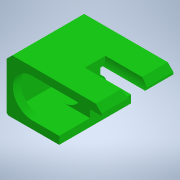
# Autodesk Inventor part: Y-linear bearing shroud secondary
Saved by Autodesk Inventor 2020.4 (Build 244396000, 396)
## iProperties
Created: 2021-02-25
Part Number: Y-linear bearing shroud secondary
Material: ABS Plastic
Document SubType Name: Modeling
Designer: AOB
Mass: 6.2455 g
Surface Area: 48.8239 cm^2
Volume: 5.89199 cm^3
Density: 1.06 g/cm^3
Appearance: Dark Green
Author: AOB
Autodesk Inventor part; units mm, degrees
ref_plane "YZ Plane" through (0, 0, 0) normal (1, 0, 0) x (0, 1, 0)
ref_plane "XZ Plane" through (0, 0, 0) normal (0, 1, 0) x (-1, 0, 0)
sketch "Sketch1" plane through (0, 0, 0) normal (0, 0, 1) x (1, 0, 0)
  line L0 (-9.0445, -10.4807) -> (0.0261, -10.458)
  line L1 (-10, 8.3388) -> (-10, 0)
  line L2 (-10, 0) -> (-9.9763, -9.4855)
  line L3 (27, 8.3389) -> (27, 7.5575)
  line L4 (24.782, 10.5568) -> (27, 8.3389)
  line L5 (-7.782, 10.5568) -> (-10, 8.3388)
  arc A0 (-9.9763, -9.4855) -> (-8.9738, -10.483) centre (-8.9763, -9.483) ccw
  arc A1 (-0.0188, 7.5552) -> (-0.012, -7.4448) centre (-0.0154, 0.0552) ccw
  line L6 (5, 7.5575) -> (-0.0188, 7.5552)
  line L7 (0.0261, -10.458) -> (7.5, -10.458)
  line L8 (7.5, 0.0187) -> (10.5, 0.0187) construction
  line L9 (10.5, -10.458) -> (7.5, -10.458)
  line L10 (-0.012, -7.4448) -> (10.5, -7.4448)
  line L11 (10.5, -7.4448) -> (10.5, -10.458)
  line L12 (-7.782, 10.5568) -> (24.782, 10.5568)
  line L13 (27, 7.5575) -> (5, 7.5575)
  point P0 (0, 0)
  point P1 (-10.0264, 10.5568)
  point P2 (27, 10.5568)
  point P3 (-10, 10.5568)
  dimension "d0" = 2.218
  dimension "d47" = 27
  constraints: 28 end point, 5 point on circle, 3 point on line, 2 centre point, 2 horizontal, 2 perpendicular, 2 tangent, 1 parallel, 1 vertical
  measures "d0" distance of L5.start point (-10, 10.557)
  measures "d47" distance from line of point (0, 0) L3
extrude "Extrusion1" add sketch "Sketch1" along normal blind 3
sketch "Sketch2" plane through (0, 0, 0) normal (0, 0, -1) x (-1, 0, 0)
  line L0 (-27, 7.5575) -> (-27, 8.3389)
  line L1 (-27, 7.5575) -> (-27, 8.3389)
  line L2 (-27, 8.3389) -> (-24.782, 10.5568)
  line L3 (-27, 8.3389) -> (-24.782, 10.5568)
  line L4 (-24.782, 10.5568) -> (7.782, 10.5568)
  line L5 (-24.782, 10.5568) -> (7.782, 10.5568)
  line L6 (7.782, 10.5568) -> (10, 8.3388)
  line L7 (9.0445, -10.4807) -> (-0.0261, -10.458)
  arc A0 (0.012, -7.4448) -> (0.0188, 7.5552) centre (0.0154, 0.0552) ccw
  line L8 (7.5154, 0.0552) -> (7.5154, 7.5518)
  line L9 (7.5154, -7.4482) -> (7.5154, 0.0552)
  line L10 (0.012, -7.4448) -> (7.5154, -7.4482)
  line L11 (-10.5, -7.4448) -> (-10.5, -10.458)
  line L12 (-10.5, -7.4448) -> (0.012, -7.4448) projected
  line L13 (-10.5, -7.4448) -> (0.012, -7.4448)
  line L14 (-5, 7.5575) -> (-27, 7.5575)
  line L15 (0.0188, 7.5552) -> (-5, 7.5575)
  line L16 (10, 0) -> (9.9763, -9.4855)
  arc A1 (9.0445, -10.4807) -> (9.9763, -9.4855) centre (8.9763, -9.483) ccw
  line L17 (10, 8.3388) -> (10, 0)
  line L18 (7.5154, 7.5518) -> (0.0188, 7.5552)
  line L19 (-0.0261, -10.458) -> (-10.5, -10.458)
  point P0 (0, 0)
  point P1 (7.5, -10.4768)
  point P2 (7.5154, -7.4448)
  constraints: 38 end point, 5 point on circle, 4 collinear, 3 tangent, 3 vertical, 2 centre point, 2 point on line
extrude "Extrusion2" add sketch "Sketch2" along normal blind 11 contours L0 L2 L4 L6 L17 L16 A1 L7 L19 L11 L12 L10 L9 L8 L18 L15 L14
ref_plane "Work Plane1" through (0, 0, -11) normal (0, 0, -1) x (-1, 0, 0)
sketch "Sketch4" plane through (0, 0, -11) normal (0, 0, -1) x (-1, 0, 0)
  line L0 (7.5154, 7.5518) -> (7.5154, -7.4482) projected
  line L1 (7.5154, 0.0552) -> (7.5154, 7.5125)
  line L2 (-7.4813, 7.5125) -> (-7.4812, 7.5187)
  line L3 (0.0341, 7.5) -> (7.5154, 7.5125)
  line L4 (-27, 7.5575) -> (-5, 7.5575) projected
  line L5 (-5, 7.5575) -> (7.5154, 7.5518) projected
  arc A0 (7.5154, 0.0552) -> (0.0188, 7.5552) centre (0.0154, 0.0552) ccw projected
  point P0 (0, 0)
  point P1 (7.5, -10.4768)
  point P2 (7.5154, -7.4482)
  point P3 (0.9117, 7.5014)
  constraints: 6 end point, 1 vertical, 1 other
extrude "Extrusion4" add sketch "Sketch4" against normal blind 2 contours L0 A0 L3
mirror "Mirror1" about plane through (0, 0, -11) normal (0, 0, -1) of "Extrusion1", "Extrusion2", "Extrusion4"
sketch "Sketch6" plane through (0, 0, -11) normal (0, 0, -1) x (-1, 0, 0)
  line L0 (-10.5, -7.4448) -> (0.012, -7.4448) projected
  arc A0 (0.0188, 7.5552) -> (7.5154, 0.0518) centre (0.0154, 0.0552) ccw
  line L1 (-10.5, -10.458) -> (-10.5, -7.4448) projected
  line L2 (0.012, -7.4448) -> (-10.5, -7.4448)
  line L3 (-10.5, -7.4448) -> (-10.5, 7.56)
  arc A1 (0.012, -7.4448) -> (0.0188, 7.5552) centre (0.0154, 0.0552) ccw
  line L4 (0.0188, 7.5552) -> (-26.9847, 7.5675)
  line L5 (-10.5, 7.56) -> (0.0188, 7.5552)
  arc A2 (0.012, -7.4448) -> (0.0188, 7.5552) centre (0.0154, 0.0552) ccw projected
  line L6 (-11.9846, 7.5606) -> (-11.9846, 0.9346) construction
  line L7 (-10.5, 0.9516) -> (-7.4308, 0.9516)
  line L8 (-8.9573, 7.5593) -> (-8.9573, 3.4333) construction
  line L9 (-10.5, 3.4516) -> (-6.6715, 3.4516)
  line L10 (-10.5, 3.4516) -> (-10.5, 5.4516)
  line L11 (-10.5, 5.4516) -> (-5.1931, 5.4516)
  line L12 (-10.5, -1.5484) -> (-10.5, 0.9516)
  line L13 (-5.1931, 5.4516) -> (-5.1931, -5.3412)
  line L14 (-10.5, 0.9516) -> (-10.5, -1.5484)
  line L15 (-10.5, 0.9516) -> (-10.5, -1.5484) construction
  spline S0 degree 1 poles (-10.5, 0.9516) (-10.5, -1.5484) knots 1 1 2 2
  line L16 (-10.5, -1.5484) -> (-7.3112, -1.5484)
  line L17 (7.5154, -7.4482) -> (7.5154, 0.0552) projected
  line L18 (0.012, -7.4448) -> (7.5154, -7.4482)
  arc A3 (0.012, -7.4448) -> (7.5154, 0.0552) centre (0.0154, 0.0552) ccw projected
  point P0 (-10.5, 7.56)
  dimension "d26" = 6.626
  dimension "d27" = 4.126
  dimension "d28" = 2
  dimension "d35" = 2.5
  dimension "d41" = 2.5
  constraints: 30 end point, 12 point on circle, 6 point on line, 5 horizontal, 4 collinear, 3 vertical, 2 centre point, 1 coincident, 1 perpendicular, 1 tangent, 3 other
  measures "d26" distance of L6.start L6.end
  measures "d27" distance of L8.start L8.end
  measures "d28" distance of L9.start L10.end
  measures "d35" distance of L7.start L12.start
  measures "d41" distance between parallel lines of L7 L9
revolve "Revolution1" add sketch "Sketch6" angle 360 about axis through (10.5, 0.9516, -11) along (-1, 0, 0) contours A0 L9 L3 L11
extrude "Extrusion3" cut sketch "Sketch6" against normal mid plane 11 contours A0 L13
extrude "Extrusion5" add sketch "Sketch6" along normal mid plane 4 contours L3 L16 A0 L0 | L11 L3 L4 A0 | A0 L9 L3 L11
sketch "Sketch7" plane through (10.5, -10.458, 3) normal (1, 0, 0) x (0, 0, -1)
  circle A0 centre (14, 20.6966) radius 4.0015
  line L0 (14, 13.9097) -> (14, 14.9097)
  line L1 (0, 18.7969) -> (28, 18.7969) projected
  line L2 (14, 14.9097) -> (14, 20.6966)
  point P0 (14, 8.9097)
  dimension "d43" = 8.003
  dimension "d48" = 1
  dimension "d49" = 5.7869
  constraints: 4 end point, 1 centre point, 1 coincident, 1 perpendicular, 1 point on line, 1 vertical alignment
  measures "d43" diameter of A0
  measures "d48" distance of L0.start L0.end
  measures "d49" distance of L0.end L2.end
extrude "Extrusion10" cut sketch "Sketch7" along normal up to surface (16.5 mm away)
body "Solid1"
